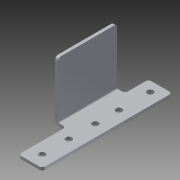
# Autodesk Inventor part: Back Brace Mount V2
Saved by Autodesk Inventor 2013 (Build 170138000, 138)
## iProperties
Created: 2013-02-10
Part Number: Back Brace Mount V2
Material: Aluminum 6061
Document SubType Name: Sheet Metal
Designer: Moses
Density: 2.71 g/cm^3
Sheet Metal Rule: Default
Flat Pattern Width: 10.2081 cm
Flat Pattern Length: 13.97 cm
Flat Pattern Area: 142.607 cm^2
Sheet Metal Width: 4.019 in
Sheet Metal Length: 5.500 in
Sheet Metal Area: 22.104 in^2
Mass: 61.9104 g
Surface Area: 171.491 cm^2
Volume: 22.8452 cm^3
Author: Moses
Autodesk Inventor part; units mm, degrees
ref_plane "YZ Plane" through (0, 0, 0) normal (1, 0, 0) x (0, 1, 0)
ref_plane "XZ Plane" through (0, 0, 0) normal (0, 1, 0) x (-1, 0, 0)
ref_plane "XY Plane" through (0, 0, 0) normal (0, 0, 1) x (1, 0, 0)
sketch "Sketch1" plane through (0, 0, 0) normal (0, 1, 0) x (-1, 0, 0)
  line L0 (0, 0) -> (25.4, 0)
  line L1 (25.4, 0) -> (25.4, 139.7)
  line L2 (25.4, 139.7) -> (0, 139.7)
  line L3 (0, 139.7) -> (0, 0)
  line L4 (12.7, 139.7) -> (12.7, 0) construction
  circle A0 centre (12.7, 127) radius 3.302
  circle A1 centre (12.7, 98.425) radius 3.302
  circle A2 centre (12.7, 69.85) radius 3.302
  circle A3 centre (12.7, 44.45) radius 3.302
  circle A4 centre (12.7, 10.795) radius 3.302
  line L5 (25.4, 88.9) -> (36.9316, 88.9)
  line L6 (36.9316, 88.9) -> (36.9316, 25.4)
  line L7 (36.9316, 25.4) -> (25.4, 25.4)
  dimension "d0" = 25.4
  dimension "d1" = 139.7
  dimension "d2" = 12.7
  dimension "d3" = 28.575
  dimension "d4" = 28.575
  dimension "d5" = 25.4
  dimension "d6" = 33.655
  dimension "d7" = 6.604
  dimension "d8" = 63.5
  dimension "d9" = 11.5316
  dimension "d10" = 50.8
  measures "d0" distance of L0.start L0.end
  measures "d1" distance of L2.end L0.start
  measures "d2" distance from line of L2 A0.centre
  measures "d3" distance of A1.centre A0.centre
  measures "d4" distance of A2.centre A1.centre
  measures "d5" distance of A3.centre A2.centre
  measures "d6" distance of A4.centre A3.centre
  measures "d7" diameter of A0
  measures "d8" distance of L5.end L6.end
  measures "d9" distance of L5.start L5.end
  measures "d10" distance from line of L5 L2.end
extrude "Plate1" add sketch "Sketch1" along normal blind 3.175
sketch "Sketch2" plane through (-33.7566, 0, 88.9) normal (-1, 0, 0) x (0, -1, 0)
  line L0 (0, -63.5) -> (0, 0)
  line L1 (0, 0) -> (-69.85, 0)
  line L2 (-69.85, 0) -> (-69.85, -63.5)
  line L3 (-69.85, -63.5) -> (0, -63.5)
  constraints: 6 end point, 1 horizontal, 1 perpendicular, 1 vertical
edge flange "Flange1" height 69.85 angle 90 thickness 3.175 bend radius 1.27 thickness toward (-1, 0, 0) relief straight relief width 3.175 relief depth 1.5875 edges at (-36.9316, 3.175, 57.15) wall of the first edge with corners at (-33.7566, 0, 25.4) (-33.7566, 0, 88.9) (-33.7566, 69.85, 88.9) (-33.7566, 69.85, 25.4)
bend "Bend1"
corner "Corner1"
fillet "Corner Round1" radius 3.175 8 edges at (0, 1.5875, 139.7) (-25.4, 1.5875, 139.7) (-25.4, 1.5875, 88.9) (-25.4, 1.5875, 25.4) (-25.4, 1.5875, 0) (0, 1.5875, 0) (-35.3441, 69.85, 88.9) (-35.3441, 69.85, 25.4)
sketch "Sketch3" plane through (-33.7566, 4.445, 88.9) normal (1, 0, 0) x (0, 0, -1)
  circle A0 centre (14.2494, 53.419) radius 3.175 construction
  circle A1 centre (49.2506, 53.419) radius 3.175 construction
  line L0 (57.15, 69.9798) -> (57.15, 47.069) construction
  line L1 (6.35, 69.9798) -> (57.15, 69.9798) construction
  line L2 (6.35, 47.069) -> (6.35, 69.9798) construction
  line L3 (6.35, 47.069) -> (57.15, 47.069) construction
  circle A2 centre (14.2494, 53.419) radius 3.3782
  circle A3 centre (49.2506, 53.419) radius 3.3782
  line L4 (60.325, 65.405) -> (3.175, 65.405) projected
  line L5 (0, 62.23) -> (0, 0) projected
  line L6 (0, 0) -> (63.5, 0) projected
  line L7 (63.5, 62.23) -> (63.5, 0) projected
  circle A4 centre (12.7, 12.7) radius 7.9375
  circle A5 centre (12.7, 38.1) radius 7.9375
  circle A6 centre (50.8, 12.7) radius 7.9375
  circle A7 centre (50.8, 38.1) radius 7.9375
  line L8 (12.7, 12.7) -> (50.8, 12.7) construction
  line L9 (31.75, 65.405) -> (31.75, 0) construction
  circle A8 centre (31.75, 25.4) radius 7.9375
  line L10 (50.8, 38.1) -> (50.8, 12.7) construction
  line L11 (31.75, 25.4) -> (50.8, 25.4) construction
  point P0 (88.9, -4.445)
  point P1 (31.75, 12.7)
  dimension "d23" = 6.7564
  dimension "d25" = 6.7564
  dimension "d28" = 15.875
  dimension "d31" = 25.4
  dimension "d34" = 38.1
  dimension "d37" = 12.7
  dimension "d38" = 15.875
  constraints: 8 end point, 7 centre point, 4 midpoint, 2 coincident, 2 horizontal, 2 perpendicular, 2 point on line, 1 vertical, 6 other
  measures "d23" diameter of A2
  measures "d25" diameter of A3
  measures "d28" diameter of A4
  measures "d31" distance of L8.start A5.centre
  measures "d34" distance of L8.start L8.end
  measures "d37" distance from line of L6 L8.start
  measures "d38" diameter of A8
extrude "Cut1" cut sketch "Sketch3" against normal blind 3.175
equation "\"d4\" = d3"
equation "\"d26\" = Thickness"
equation "\"d12\" = BendReliefWidth"
equation "\"d13\" = BendReliefDepth"
equation "\"d14\" = MinimumRemnant"
equation "\"d15\" = BendRadius"
equation "\"d19\" = CornerReliefSize"
equation "\"d20\" = GapSize"
equation "\"d21\" = JacobiRadiusSize"
equation "\"BendRadius\" = Thickness"
equation "\"BendReliefWidth\" = Thickness"
equation "\"BendReliefDepth\" = 0.5 * Thickness"
equation "\"CornerReliefSize\" = 4 * Thickness"
equation "\"MinimumRemnant\" = 2 * Thickness"
equation "\"TransitionRadius\" = BendRadius"
equation "\"JacobiRadiusSize\" = BendRadius"
equation "\"GapSize\" = Thickness"
equation "\"d11\" = BendRadius"
equation "\"Thickness\" = 3.175"
body "Solid1"
